acrylic_topcover_v3 (Autodesk Fusion 360 design; units mm, degrees)
Autodesk Fusion 360 part; units mm, degrees
sketch "Sketch1" plane through (0, 0, 0) normal (0, 1, 0) x (1, 0, 0)
  line L0 (431.8, 212.7255) -> (215.9, 212.7255) construction
  line L1 (0, 0) -> (215.9, 0) construction
  circle A0 centre (238.9, 201.7255) radius 3
  line L2 (215.9, 212.7255) -> (215.9, 106.363) construction
  line L3 (0, 106.363) -> (215.9, 106.363) construction
  line L4 (431.8, 0) -> (431.8, 106.3625) construction
  circle A1 centre (23, 95.3625) radius 3
  line L5 (-1, 213.7255) -> (-1, 91.8373)
  circle A2 centre (23, 12) radius 3
  circle A3 centre (193.9, 95.3625) radius 3
  line L6 (193.9, 118.363) -> (193.9, 201.7255) construction
  line L7 (193.9, 95.3625) -> (23, 95.3625) construction
  line L8 (238.9, 201.7255) -> (238.9, 118.363) construction
  line L9 (0, 212.7255) -> (0, 106.363) construction
  line L10 (409.8, 95.3625) -> (238.9, 95.3625) construction
  line L11 (431.8, 106.3625) -> (215.9, 106.3625) construction
  line L12 (409.8, 201.7255) -> (238.9, 201.7255) construction
  line L13 (208.9, 213.7255) -> (-1, 213.7255)
  line L14 (23, 118.363) -> (193.9, 118.363) construction
  line L15 (0, 106.3625) -> (0, 0) construction
  circle A4 centre (23, 201.7255) radius 3
  circle A5 centre (193.9, 201.7255) radius 3
  line L16 (409.8, 118.363) -> (409.8, 201.7255) construction
  line L17 (215.9, 106.3625) -> (215.9, 0) construction
  line L18 (208.9, -1) -> (432.8, -1)
  circle A6 centre (409.8, 12) radius 3
  line L19 (431.8, 106.363) -> (431.8, 212.7255) construction
  line L20 (432.8, 116.8753) -> (432.8, 213.7255)
  line L21 (409.8, 12) -> (409.8, 95.3625) construction
  line L22 (238.9, 12) -> (409.8, 12) construction
  line L23 (215.9, 0) -> (215.9, 106.3625) construction
  circle A7 centre (238.9, 12) radius 3
  circle A8 centre (193.9, 12) radius 3
  line L24 (-1, 91.8373) -> (-1, -1)
  line L25 (193.9, 12) -> (193.9, 95.3625) construction
  circle A9 centre (409.8, 201.7255) radius 3
  circle A10 centre (193.9, 118.363) radius 3
  line L26 (23, 12) -> (193.9, 12) construction
  circle A11 centre (23, 118.363) radius 3
  line L27 (193.9, 201.7255) -> (23, 201.7255) construction
  circle A12 centre (238.9, 95.3625) radius 3
  line L28 (23, 201.7255) -> (23, 118.363) construction
  line L29 (23, 95.3625) -> (23, 12) construction
  line L30 (432.8, 213.7255) -> (208.9, 213.7255)
  line L31 (238.9, 95.3625) -> (238.9, 12) construction
  line L32 (215.9, 106.3625) -> (0, 106.3625) construction
  circle A13 centre (409.8, 118.363) radius 3
  line L33 (-1, -1) -> (208.9, -1)
  circle A14 centre (409.8, 95.3625) radius 3
  line L34 (238.9, 118.363) -> (409.8, 118.363) construction
  line L35 (215.9, 106.363) -> (215.9, 212.7255) construction
  circle A15 centre (238.9, 118.363) radius 3
  line L36 (432.8, -1) -> (432.8, 116.8753)
  line L37 (215.9, 212.7255) -> (0, 212.7255) construction
  line L38 (215.9, 106.363) -> (431.8, 106.363) construction
  line L39 (215.9, 0) -> (431.8, 0) construction
  point P0 (215.9, 106.363)
  point P1 (0, 106.363)
  point P2 (215.9, 0)
  dimension "d3" = 215.9
  dimension "d4" = 106.363
  dimension "d23" = 1
  dimension "d6" = 1
  dimension "d7" = 106.3625
  dimension "d8" = 215.9
  dimension "d9" = 23
  dimension "d10" = 11
  dimension "d11" = 12
  dimension "d12" = 22
  dimension "d13" = 6
  dimension "d14" = 6
  dimension "d15" = 6
  dimension "d16" = 6
  constraint horizontal L1
  constraint vertical L23
  constraint horizontal L32
  constraint vertical L15
  constraint coincident L1.start L15.end
  constraint horizontal L26
  constraint vertical L25
  constraint horizontal L7
  constraint vertical L29
  constraint coincident A1.centre L7.end
  constraint coincident A2.centre L26.start
  constraint coincident A8.centre L25.start
  constraint coincident A3.centre L7.start
  constraint coincident L5.end L24.start
  constraint coincident L20.start L36.end
  measures "d7" distance of L15.start L1.start
  measures "d8" distance of P2 L1.start
  measures "d9" distance of L15 L29
  measures "d10" distance of L7 L32
  measures "d11" distance of L1 L26
  measures "d12" distance of L23 L25
  measures "d13" diameter of A1
  measures "d14" diameter of A2
  measures "d15" diameter of A3
  measures "d16" diameter of A8
extrude "Extrude1" add sketch "Sketch1" along normal blind 6
sketch "Sketch2" plane through (0, 6, 0) normal (0, 1, 0) x (-1, 0, 0)
  circle A0 centre (-409.8, -201.7255) radius 3
  circle A1 centre (-238.9, -12) radius 3
  circle A2 centre (-193.9, -12) radius 3
  circle A3 centre (-193.9, -95.3625) radius 3
  circle A4 centre (-193.9, -201.7255) radius 3
  circle A5 centre (-409.8, -12) radius 3
  circle A6 centre (-23, -201.7255) radius 3
  circle A7 centre (-23, -118.363) radius 3
  circle A8 centre (-23, -12) radius 3
  circle A9 centre (-238.9, -201.7255) radius 3
  circle A10 centre (-23, -95.3625) radius 3
  circle A11 centre (-193.9, -118.363) radius 3
  circle A12 centre (-409.8, -118.363) radius 3
  circle A13 centre (-238.9, -118.363) radius 3
  circle A14 centre (-409.8, -95.3625) radius 3
  circle A15 centre (-238.9, -95.3625) radius 3
  line L0 (-432.8, 1) -> (-432.8, -116.8753)
  line L1 (-432.8, -116.8753) -> (-432.8, -213.7255)
  line L2 (-432.8, -213.7255) -> (1, -213.7255)
  line L3 (1, -213.7255) -> (1, -91.8373)
  line L4 (1, -91.8373) -> (1, 1)
  line L5 (1, 1) -> (-432.8, 1)
  line L6 (-99, -165.7255) -> (-332.8, -165.7255) construction
  line L7 (-332.8, -47) -> (-99, -47) construction
  line L8 (-99, -47) -> (-99, -165.7255) construction
  arc A16 (-100.5875, -175.7255) -> (-97.4125, -175.7255) centre (-99, -175.7255) ccw
  arc A17 (-97.4125, -155.7255) -> (-100.5875, -155.7255) centre (-99, -155.7255) ccw
  line L9 (-99, -155.7255) -> (-99, -175.7255) construction
  arc A18 (-89, -167.313) -> (-89, -164.138) centre (-89, -165.7255) ccw
  arc A19 (-109, -164.138) -> (-109, -167.313) centre (-109, -165.7255) ccw
  line L10 (-109, -165.7255) -> (-89, -165.7255) construction
  arc A20 (-97.4125, -37) -> (-100.5875, -37) centre (-99, -37) ccw
  line L11 (-99, -37) -> (-99, -57) construction
  line L12 (-109, -47) -> (-89, -47) construction
  arc A21 (-89, -48.5875) -> (-89, -45.4125) centre (-89, -47) ccw
  arc A22 (-100.5875, -57) -> (-97.4125, -57) centre (-99, -57) ccw
  arc A23 (-109, -45.4125) -> (-109, -48.5875) centre (-109, -47) ccw
  arc A24 (-322.8, -167.313) -> (-322.8, -164.138) centre (-322.8, -165.7255) ccw
  arc A25 (-342.8, -164.138) -> (-342.8, -167.313) centre (-342.8, -165.7255) ccw
  line L13 (-332.8, -155.7255) -> (-332.8, -175.7255) construction
  arc A26 (-331.2125, -155.7255) -> (-334.3875, -155.7255) centre (-332.8, -155.7255) ccw
  arc A27 (-334.3875, -175.7255) -> (-331.2125, -175.7255) centre (-332.8, -175.7255) ccw
  line L14 (-342.8, -165.7255) -> (-322.8, -165.7255) construction
  arc A28 (-342.8, -45.4125) -> (-342.8, -48.5875) centre (-342.8, -47) ccw
  line L15 (-342.8, -47) -> (-322.8, -47) construction
  arc A29 (-322.8, -48.5875) -> (-322.8, -45.4125) centre (-322.8, -47) ccw
  arc A30 (-331.2125, -37) -> (-334.3875, -37) centre (-332.8, -37) ccw
  line L16 (-332.8, -37) -> (-332.8, -57) construction
  arc A31 (-334.3875, -57) -> (-331.2125, -57) centre (-332.8, -57) ccw
  line L17 (-332.8, -165.7255) -> (-332.8, -47) construction
  line L18 (-331.2125, -175.7255) -> (-331.2125, -169.189)
  line L19 (-329.3365, -167.313) -> (-322.8, -167.313)
  line L20 (-342.8, -167.313) -> (-336.2635, -167.313)
  arc A32 (-331.2125, -169.189) -> (-329.3365, -167.313) centre (-332.8, -165.7255) ccw
  line L21 (-322.8, -164.138) -> (-329.3365, -164.138)
  line L22 (-331.2125, -162.262) -> (-331.2125, -155.7255)
  line L23 (-334.3875, -155.7255) -> (-334.3875, -162.262)
  line L24 (-334.3875, -169.189) -> (-334.3875, -175.7255)
  line L25 (-331.2125, -164.138) -> (-332.8, -164.138)
  line L26 (-336.2635, -164.138) -> (-342.8, -164.138)
  arc A33 (-336.2635, -167.313) -> (-334.3875, -169.189) centre (-332.8, -165.7255) ccw
  arc A34 (-329.3365, -164.138) -> (-331.2125, -162.262) centre (-332.8, -165.7255) ccw
  arc A35 (-334.3875, -162.262) -> (-336.2635, -164.138) centre (-332.8, -165.7255) ccw
  line L27 (-331.2125, -57) -> (-331.2125, -50.4635)
  line L28 (-342.8, -48.5875) -> (-336.2635, -48.5875)
  line L29 (-329.3365, -48.5875) -> (-322.8, -48.5875)
  line L30 (-334.3875, -37) -> (-334.3875, -43.5365)
  line L31 (-334.3875, -50.4635) -> (-334.3875, -57)
  arc A36 (-336.2635, -48.5875) -> (-334.3875, -50.4635) centre (-332.8, -47) ccw
  arc A37 (-331.2125, -50.4635) -> (-329.3365, -48.5875) centre (-332.8, -47) ccw
  line L32 (-322.8, -45.4125) -> (-329.3365, -45.4125)
  line L33 (-336.2635, -45.4125) -> (-342.8, -45.4125)
  line L34 (-331.2125, -43.5365) -> (-331.2125, -37)
  arc A38 (-329.3365, -45.4125) -> (-331.2125, -43.5365) centre (-332.8, -47) ccw
  arc A39 (-334.3875, -43.5365) -> (-336.2635, -45.4125) centre (-332.8, -47) ccw
  line L35 (-97.4125, -57) -> (-97.4125, -50.4635)
  line L36 (-100.5875, -50.4635) -> (-100.5875, -57)
  line L37 (-109, -48.5875) -> (-102.4635, -48.5875)
  line L38 (-95.5365, -48.5875) -> (-89, -48.5875)
  arc A40 (-102.4635, -48.5875) -> (-100.5875, -50.4635) centre (-99, -47) ccw
  line L39 (-89, -45.4125) -> (-95.5365, -45.4125)
  line L40 (-102.4635, -45.4125) -> (-109, -45.4125)
  line L41 (-100.5875, -37) -> (-100.5875, -43.5365)
  line L42 (-97.4125, -43.5365) -> (-97.4125, -37)
  arc A41 (-100.5875, -43.5365) -> (-102.4635, -45.4125) centre (-99, -47) ccw
  arc A42 (-97.4125, -50.4635) -> (-95.5365, -48.5875) centre (-99, -47) ccw
  arc A43 (-95.5365, -45.4125) -> (-97.4125, -43.5365) centre (-99, -47) ccw
  line L43 (-100.5875, -155.7255) -> (-100.5875, -162.262)
  line L44 (-100.5875, -169.189) -> (-100.5875, -175.7255)
  line L45 (-109, -167.313) -> (-102.4635, -167.313)
  line L46 (-97.4125, -175.7255) -> (-97.4125, -169.189)
  line L47 (-95.5365, -167.313) -> (-89, -167.313)
  line L48 (-89, -164.138) -> (-95.5365, -164.138)
  line L49 (-102.4635, -164.138) -> (-109, -164.138)
  arc A44 (-102.4635, -167.313) -> (-100.5875, -169.189) centre (-99, -165.7255) ccw
  arc A45 (-100.5875, -162.262) -> (-102.4635, -164.138) centre (-99, -165.7255) ccw
  line L50 (-97.4125, -162.262) -> (-97.4125, -155.7255)
  arc A46 (-97.4125, -169.189) -> (-95.5365, -167.313) centre (-99, -165.7255) ccw
  arc A47 (-95.5365, -164.138) -> (-97.4125, -162.262) centre (-99, -165.7255) ccw
  point P0 (-99, -165.7255)
  point P1 (-99, -165.7255)
  point P2 (-99, -47)
  point P3 (-99, -47)
  point P4 (-332.8, -165.7255)
  point P5 (-332.8, -165.7255)
  point P6 (-332.8, -47)
  point P7 (-332.8, -47)
  dimension "d29" = 7.62
  dimension "d32" = 3.175
  dimension "d33" = 20
  dimension "d34" = 3.175
  dimension "d35" = 20
  dimension "d36" = 7.62
  dimension "d37" = 3.175
  dimension "d38" = 20
  dimension "d39" = 3.175
  dimension "d40" = 20
  dimension "d41" = 7.62
  dimension "d42" = 3.175
  dimension "d43" = 20
  dimension "d44" = 3.175
  dimension "d45" = 20
  dimension "d46" = 7.62
  dimension "d47" = 3.175
  dimension "d48" = 20
  dimension "d49" = 3.175
  dimension "d50" = 20
  dimension "d51" = 48
  dimension "d52" = 48
  dimension "d53" = 100
  dimension "d54" = 100
  constraint horizontal L6
  constraint horizontal L7
  constraint vertical L8
  constraint tangent A16 L43
  constraint tangent A16 L46
  constraint parallel L43 L46
  constraint tangent A17 L46
  constraint tangent A17 L43
  constraint vertical L9
  constraint coincident P1 P0
  constraint midpoint L9 P1
  constraint tangent A18 L45
  constraint tangent A18 L48
  constraint parallel L45 L48
  constraint tangent A19 L48
  constraint tangent A19 L45
  constraint perpendicular L10 L46
  constraint midpoint L10 P1
  constraint tangent A22 L41
  constraint tangent A22 L35
  constraint parallel L35 L41
  constraint tangent A20 L35
  constraint tangent A20 L41
  constraint vertical L11
  constraint coincident P3 P2
  constraint midpoint P3 L11
  constraint tangent A21 L37
  constraint tangent A21 L39
  constraint parallel L37 L39
  constraint tangent A23 L39
  constraint tangent A23 L37
  constraint perpendicular L12 L35
  constraint midpoint P3 L12
  constraint tangent A27 L23
  constraint tangent A27 L18
  constraint parallel L18 L23
  constraint tangent A26 L18
  constraint tangent A26 L23
  constraint vertical L13
  constraint coincident P5 P4
  constraint midpoint P5 L13
  constraint tangent A24 L20
  constraint tangent A24 L21
  constraint parallel L20 L21
  constraint tangent A25 L21
  constraint tangent A25 L20
  constraint perpendicular L14 L18
  constraint midpoint P5 L14
  constraint tangent A31 L30
  constraint tangent A31 L27
  constraint parallel L27 L30
  constraint tangent A30 L27
  constraint tangent A30 L30
  constraint vertical L16
  constraint coincident P7 P6
  constraint midpoint P7 L16
  constraint tangent A29 L28
  constraint tangent A29 L32
  constraint parallel L28 L32
  constraint tangent A28 L32
  constraint tangent A28 L28
  constraint perpendicular L15 L27
  constraint midpoint P7 L15
  constraint perpendicular L7 L17
  constraint coincident L24.start L23
  constraint collinear L19 L20
  constraint coincident L20.end A32
  constraint concentric A32 A34
  constraint collinear L21 L25
  constraint collinear L23 L24
  constraint coincident L13 L25.end
  constraint collinear L25 L26
  constraint coincident L23.end A34
  constraint concentric A33 A34
  constraint concentric A34 A35
  constraint coincident L27.end A36
  constraint coincident L29.start A36
  constraint collinear L28 L29
  constraint collinear L30 L31
  constraint coincident L33.start L32
  constraint concentric A36 A37
  constraint concentric A37 A38
  constraint collinear L32 L33
  constraint coincident L30.end A38
  constraint concentric A38 A39
  constraint collinear L36 L41
  constraint collinear L37 L38
  constraint coincident L37.end A42
  constraint concentric A40 A42
  constraint coincident L40.start L39
  constraint collinear L39 L40
  constraint coincident L41.end A42
  constraint concentric A41 A42
  constraint coincident L39.end A42
  constraint concentric A42 A43
  constraint collinear L43 L44
  constraint coincident L45.end A46
  constraint collinear L48 L49
  constraint concentric A44 A46
  constraint coincident L43.end A46
  constraint concentric A45 A46
  constraint coincident L48.end A46
  constraint concentric A46 A47
  measures "d29" diameter of A46
  measures "d32" distance of L43 L46
  measures "d33" distance of A17.centre A16.centre
  measures "d34" distance of L45 L48
  measures "d35" distance of A19.centre A18.centre
  measures "d36" diameter of A42
  measures "d37" distance of L35 L41
  measures "d38" distance of A20.centre L11.end
  measures "d39" distance of L37 L39
  measures "d40" distance of L12.end L12.start
  measures "d41" diameter of A32
  measures "d42" distance of L18 L23
  measures "d43" distance of L13.end L13.start
  measures "d44" distance of L20 L21
  measures "d45" distance of A24.centre A25.centre
  measures "d46" diameter of A36
  measures "d47" distance of L27 L30
  measures "d48" distance of L16.end A30.centre
  measures "d49" distance of L28 L32
  measures "d50" distance of A28.centre L15.end
  measures "d51" distance of L2 L6
  measures "d52" distance of L5 L7
  measures "d53" distance of L1 L17
  measures "d54" distance of L4 L8
extrude "Extrude2" [suppressed]
sketch "Sketch3" plane through (0, 6, 0) normal (0, 1, 0) x (-1, 0, 0)
  line L0 (-342.8, -45.4125) -> (-336.2635, -45.4125)
  arc A0 (-334.3875, -43.5365) -> (-336.2635, -45.4125) centre (-332.8, -47) ccw
  line L1 (-334.3875, -43.5365) -> (-334.3875, -37)
  arc A1 (-331.2125, -37) -> (-334.3875, -37) centre (-332.8, -37) ccw
  line L2 (-331.2125, -37) -> (-331.2125, -43.5365)
  arc A2 (-329.3365, -45.4125) -> (-331.2125, -43.5365) centre (-332.8, -47) ccw
  line L3 (-329.3365, -45.4125) -> (-322.8, -45.4125)
  arc A3 (-322.8, -48.5875) -> (-322.8, -45.4125) centre (-322.8, -47) ccw
  line L4 (-322.8, -48.5875) -> (-329.3365, -48.5875)
  arc A4 (-331.2125, -50.4635) -> (-329.3365, -48.5875) centre (-332.8, -47) ccw
  line L5 (-331.2125, -50.4635) -> (-331.2125, -57)
  arc A5 (-334.3875, -57) -> (-331.2125, -57) centre (-332.8, -57) ccw
  line L6 (-334.3875, -57) -> (-334.3875, -50.4635)
  arc A6 (-336.2635, -48.5875) -> (-334.3875, -50.4635) centre (-332.8, -47) ccw
  line L7 (-336.2635, -48.5875) -> (-342.8, -48.5875)
  arc A7 (-342.8, -45.4125) -> (-342.8, -48.5875) centre (-342.8, -47) ccw
  line L8 (-97.4125, -37) -> (-97.4125, -43.5365)
  arc A8 (-95.5365, -45.4125) -> (-97.4125, -43.5365) centre (-99, -47) ccw
  line L9 (-95.5365, -45.4125) -> (-89, -45.4125)
  arc A9 (-89, -48.5875) -> (-89, -45.4125) centre (-89, -47) ccw
  line L10 (-89, -48.5875) -> (-95.5365, -48.5875)
  arc A10 (-97.4125, -50.4635) -> (-95.5365, -48.5875) centre (-99, -47) ccw
  line L11 (-97.4125, -50.4635) -> (-97.4125, -57)
  arc A11 (-100.5875, -57) -> (-97.4125, -57) centre (-99, -57) ccw
  line L12 (-100.5875, -57) -> (-100.5875, -50.4635)
  arc A12 (-102.4635, -48.5875) -> (-100.5875, -50.4635) centre (-99, -47) ccw
  line L13 (-102.4635, -48.5875) -> (-109, -48.5875)
  arc A13 (-109, -45.4125) -> (-109, -48.5875) centre (-109, -47) ccw
  line L14 (-109, -45.4125) -> (-102.4635, -45.4125)
  arc A14 (-100.5875, -43.5365) -> (-102.4635, -45.4125) centre (-99, -47) ccw
  line L15 (-100.5875, -43.5365) -> (-100.5875, -37)
  arc A15 (-97.4125, -37) -> (-100.5875, -37) centre (-99, -37) ccw
  line L16 (-342.8, -164.138) -> (-336.2635, -164.138)
  arc A16 (-334.3875, -162.262) -> (-336.2635, -164.138) centre (-332.8, -165.7255) ccw
  line L17 (-334.3875, -162.262) -> (-334.3875, -155.7255)
  arc A17 (-331.2125, -155.7255) -> (-334.3875, -155.7255) centre (-332.8, -155.7255) ccw
  line L18 (-331.2125, -155.7255) -> (-331.2125, -162.262)
  arc A18 (-329.3365, -164.138) -> (-331.2125, -162.262) centre (-332.8, -165.7255) ccw
  line L19 (-329.3365, -164.138) -> (-322.8, -164.138)
  arc A19 (-322.8, -167.313) -> (-322.8, -164.138) centre (-322.8, -165.7255) ccw
  line L20 (-322.8, -167.313) -> (-329.3365, -167.313)
  arc A20 (-331.2125, -169.189) -> (-329.3365, -167.313) centre (-332.8, -165.7255) ccw
  line L21 (-331.2125, -169.189) -> (-331.2125, -175.7255)
  arc A21 (-334.3875, -175.7255) -> (-331.2125, -175.7255) centre (-332.8, -175.7255) ccw
  line L22 (-334.3875, -175.7255) -> (-334.3875, -169.189)
  arc A22 (-336.2635, -167.313) -> (-334.3875, -169.189) centre (-332.8, -165.7255) ccw
  line L23 (-336.2635, -167.313) -> (-342.8, -167.313)
  arc A23 (-342.8, -164.138) -> (-342.8, -167.313) centre (-342.8, -165.7255) ccw
  line L24 (-97.4125, -155.7255) -> (-97.4125, -162.262)
  arc A24 (-95.5365, -164.138) -> (-97.4125, -162.262) centre (-99, -165.7255) ccw
  line L25 (-95.5365, -164.138) -> (-89, -164.138)
  arc A25 (-89, -167.313) -> (-89, -164.138) centre (-89, -165.7255) ccw
  line L26 (-89, -167.313) -> (-95.5365, -167.313)
  arc A26 (-97.4125, -169.189) -> (-95.5365, -167.313) centre (-99, -165.7255) ccw
  line L27 (-97.4125, -169.189) -> (-97.4125, -175.7255)
  arc A27 (-100.5875, -175.7255) -> (-97.4125, -175.7255) centre (-99, -175.7255) ccw
  line L28 (-100.5875, -175.7255) -> (-100.5875, -169.189)
  arc A28 (-102.4635, -167.313) -> (-100.5875, -169.189) centre (-99, -165.7255) ccw
  line L29 (-102.4635, -167.313) -> (-109, -167.313)
  arc A29 (-109, -164.138) -> (-109, -167.313) centre (-109, -165.7255) ccw
  line L30 (-109, -164.138) -> (-102.4635, -164.138)
  arc A30 (-100.5875, -162.262) -> (-102.4635, -164.138) centre (-99, -165.7255) ccw
  line L31 (-100.5875, -162.262) -> (-100.5875, -155.7255)
  arc A31 (-97.4125, -155.7255) -> (-100.5875, -155.7255) centre (-99, -155.7255) ccw
  circle A32 centre (-409.8, -201.7255) radius 3
  circle A33 centre (-238.9, -12) radius 3
  circle A34 centre (-193.9, -12) radius 3
  circle A35 centre (-193.9, -95.3625) radius 3
  circle A36 centre (-193.9, -201.7255) radius 3
  circle A37 centre (-409.8, -12) radius 3
  circle A38 centre (-23, -201.7255) radius 3
  circle A39 centre (-23, -118.363) radius 3
  circle A40 centre (-23, -12) radius 3
  circle A41 centre (-238.9, -201.7255) radius 3
  circle A42 centre (-23, -95.3625) radius 3
  circle A43 centre (-193.9, -118.363) radius 3
  circle A44 centre (-409.8, -118.363) radius 3
  circle A45 centre (-238.9, -118.363) radius 3
  circle A46 centre (-409.8, -95.3625) radius 3
  circle A47 centre (-238.9, -95.3625) radius 3
  line L32 (-432.8, 1) -> (-432.8, -116.8753)
  line L33 (-432.8, -116.8753) -> (-432.8, -213.7255)
  line L34 (-432.8, -213.7255) -> (1, -213.7255)
  line L35 (1, -213.7255) -> (1, -91.8373)
  line L36 (1, -91.8373) -> (1, 1)
  line L37 (1, 1) -> (-432.8, 1)
  line L38 (-434.9957, -207.7255) -> (-434.9957, -213.7255)
  line L39 (-434.9957, 1) -> (-428.9957, 1)
  line L40 (-217.9, -213.7255) -> (-217.9, -219.7255)
  circle A48 centre (-193.9, -118.363) radius 3
  circle A49 centre (-23, -201.7255) radius 3
  circle A50 centre (-23, -118.363) radius 3
  circle A51 centre (-193.9, -12) radius 3
  line L41 (-211.9, 7) -> (-211.9, 1)
  circle A52 centre (-409.8, -95.3625) radius 3
  line L42 (1, -5) -> (1, 1)
  line L43 (7, -207.7255) -> (1, -207.7255)
  line L44 (1, 1) -> (-434.9957, 1)
  line L45 (1, -213.7255) -> (1, -97.8373)
  line L46 (-434.9957, 1) -> (-434.9957, -24)
  line L47 (-434.9957, -24) -> (-251.0957, -24)
  circle A53 centre (-23, -95.3625) radius 3
  circle A54 centre (-23, -12) radius 3
  circle A55 centre (-193.9, -201.7255) radius 3
  circle A56 centre (-193.9, -95.3625) radius 3
  line L48 (1, -97.8373) -> (1, 1)
  line L49 (1, -213.7255) -> (-5, -213.7255)
  line L50 (-217.9, -219.7255) -> (-211.9, -219.7255)
  line L51 (7, -5) -> (1, -5)
  circle A57 centre (-409.8, -201.7255) radius 3
  line L52 (-440.9957, -207.7255) -> (-434.9957, -207.7255)
  line L53 (-211.9, -213.7255) -> (-217.9, -213.7255)
  circle A58 centre (-238.9, -118.363) radius 3
  line L54 (1, -219.7255) -> (1, -213.7255)
  line L55 (1, 1) -> (-5, 1)
  circle A59 centre (-238.9, -12) radius 3
  line L56 (-440.9957, -5) -> (-434.9957, -5)
  line L57 (-217.9, 7) -> (-211.9, 7)
  line L58 (1, 1) -> (7, 1)
  circle A60 centre (-409.8, -12) radius 3
  line L59 (-5, 1) -> (-5, 7)
  line L60 (-428.9957, 7) -> (-434.9957, 7)
  line L61 (-434.9957, -213.7255) -> (-428.9957, -213.7255)
  line L62 (-211.9, 1) -> (-217.9, 1)
  line L63 (-434.9957, -219.7255) -> (-434.9957, -213.7255)
  line L64 (1, -207.7255) -> (1, -213.7255)
  line L65 (-211.9, -219.7255) -> (-211.9, -213.7255)
  circle A61 centre (-409.8, -118.363) radius 3
  line L66 (-5, -219.7255) -> (1, -219.7255)
  circle A62 centre (-238.9, -201.7255) radius 3
  line L67 (-217.9, 1) -> (-217.9, 7)
  line L68 (-428.9957, -219.7255) -> (-434.9957, -219.7255)
  line L69 (7, -213.7255) -> (7, -207.7255)
  line L70 (-434.9957, -5) -> (-434.9957, 1)
  line L71 (-434.9957, -213.7255) -> (-440.9957, -213.7255)
  line L72 (-428.9957, 1) -> (-428.9957, 7)
  line L73 (7, 1) -> (7, -5)
  line L74 (-428.9957, -213.7255) -> (-428.9957, -219.7255)
  circle A63 centre (-238.9, -95.3625) radius 3
  line L75 (-434.9957, 7) -> (-434.9957, 1)
  line L76 (-440.9957, -213.7255) -> (-440.9957, -207.7255)
  line L77 (-440.9957, 1) -> (-440.9957, -5)
  line L78 (-434.9957, 1) -> (-440.9957, 1)
  line L79 (1, -213.7255) -> (7, -213.7255)
  line L80 (-5, -213.7255) -> (-5, -219.7255)
  line L81 (1, 7) -> (1, 1)
  line L82 (-5, 7) -> (1, 7)
  dimension "d57" = 6
  dimension "d58" = 6
  dimension "d59" = 6
  dimension "d60" = 6
  dimension "d61" = 6
  dimension "d62" = 6
  dimension "d63" = 6
  dimension "d64" = 6
  dimension "d65" = 6
  dimension "d66" = 6
  dimension "d67" = 6
  dimension "d68" = 6
  dimension "d69" = 6
  dimension "d70" = 6
  dimension "d71" = 6
  dimension "d72" = 6
  dimension "d73" = 6
  dimension "d74" = 6
  dimension "d75" = 6
  dimension "d76" = 6
  dimension "d77" = 212.9
  dimension "d78" = 212.9
  constraint horizontal L79
  constraint vertical L69
  constraint horizontal L43
  constraint vertical L64
  constraint coincident L34.end L35.start
  constraint horizontal L58
  constraint vertical L73
  constraint horizontal L51
  constraint vertical L42
  constraint coincident L36.end L37.start
  constraint horizontal L55
  constraint vertical L59
  constraint horizontal L82
  constraint vertical L81
  constraint horizontal L49
  constraint vertical L80
  constraint horizontal L66
  constraint vertical L54
  constraint horizontal L61
  constraint vertical L74
  constraint horizontal L68
  constraint vertical L63
  constraint horizontal L71
  constraint vertical L76
  constraint horizontal L52
  constraint vertical L38
  constraint horizontal L78
  constraint vertical L77
  constraint horizontal L56
  constraint vertical L70
  constraint coincident L39.start L44.end
  constraint horizontal L39
  constraint vertical L72
  constraint horizontal L60
  constraint vertical L75
  constraint horizontal L62
  constraint vertical L67
  constraint horizontal L57
  constraint vertical L41
  constraint coincident L41.end L44
  constraint horizontal L53
  constraint vertical L40
  constraint horizontal L50
  constraint vertical L65
  measures "d57" distance of L36.end L58.end
  measures "d58" distance of L51.start L58.end
  measures "d59" distance of L34.end L69.start
  measures "d60" distance of L43.start L69.start
  measures "d61" distance of L55.end L36.end
  measures "d62" distance of L81.start L36.end
  measures "d63" distance of L34.end L54.start
  measures "d64" distance of L54.start L66.start
  measures "d65" distance of L38.end L61.end
  measures "d66" distance of L38.end L63.start
  measures "d67" distance of L38.end L71.end
  measures "d68" distance of L38.end L38.start
  measures "d69" distance of L39.start L77.start
  measures "d70" distance of L39.start L56.end
  measures "d71" distance of L39.start L39.end
  measures "d72" distance of L39.start L60.end
  measures "d73" distance of L41.end L62.end
  measures "d74" distance of L41.start L41.end
  measures "d75" distance of L53.start L40.start
  measures "d76" distance of L53.start L50.end
  measures "d77" distance of L45 L65
  measures "d78" distance of L41 L48
equation "d28 = 0.3 in"
equation "d29 = d28"
equation "d32 = 1 in / 8"
equation "d34 = d32"
equation "d35 = d33"
equation "d36 = d28"
equation "d37 = 1 in / 8"
equation "d39 = d32"
equation "d40 = d33"
equation "d41 = d28"
equation "d42 = 1 in / 8"
equation "d44 = d32"
equation "d45 = d33"
equation "d46 = d28"
equation "d47 = 1 in / 8"
equation "d49 = d32"
equation "d50 = d33"
equation "d52 = d51"
equation "d54 = d53"
